Autodesk Fusion 360 part; units mm, degrees
(part 5 of 13)
  line L3550 (131.339, -140.663) -> (131.339, -140.663)
  line L3551 (130.416, -139.988) -> (130.432, -140.022)
  line L3552 (131.079, -140.585) -> (131.123, -140.605)
  line L3553 (129.684, -140.51) -> (129.684, -140.51)
  line L3554 (131.339, -140.663) -> (131.344, -140.664)
  line L3555 (130.303, -139.915) -> (130.371, -139.936)
  line L3556 (130.172, -140.022) -> (130.188, -139.988)
  line L3557 (128.804, -140.664) -> (129.032, -140.684)
  line L3558 (128.588, -140.606) -> (128.588, -140.606)
  line L3559 (130.732, -140.38) -> (130.733, -140.38)
  line L3560 (130.733, -140.38) -> (130.915, -140.508)
  line L3561 (131.572, -140.684) -> (131.8, -140.664)
  line L3562 (127.892, -140.022) -> (127.894, -140.027)
  line L3563 (128.192, -140.38) -> (128.192, -140.38)
  line L3564 (129.26, -140.664) -> (129.265, -140.663)
  line L3565 (127.149, -140.508) -> (127.331, -140.38)
  line L3566 (128.588, -140.606) -> (128.799, -140.663)
  line L3567 (130.732, -140.38) -> (130.732, -140.38)
  line L3568 (131.123, -140.605) -> (131.128, -140.606)
  line L3569 (135.315, -139.935) -> (135.383, -139.915)
  line L3570 (134.952, -140.38) -> (134.956, -140.377)
  line L3571 (132.911, -139.936) -> (132.956, -139.988)
  line L3572 (132.224, -140.51) -> (132.224, -140.51)
  line L3573 (133.106, -140.215) -> (133.268, -140.377)
  line L3574 (134.764, -140.51) -> (134.769, -140.508)
  line L3575 (132.578, -140.215) -> (132.71, -140.027)
  line L3576 (133.884, -140.664) -> (134.112, -140.684)
  line L3577 (130.235, -139.935) -> (130.303, -139.915)
  line L3578 (134.561, -140.605) -> (134.605, -140.585)
  line L3579 (132.972, -140.022) -> (132.972, -140.022)
  line L3580 (135.383, -139.915) -> (135.451, -139.936)
  line L3581 (134.34, -140.664) -> (134.345, -140.663)
  line L3582 (135.252, -140.022) -> (135.252, -140.022)
  line L3583 (132.712, -140.022) -> (132.728, -139.988)
  line L3584 (132.016, -140.606) -> (132.021, -140.605)
  line L3585 (130.038, -140.215) -> (130.17, -140.027)
  line L3586 (133.272, -140.38) -> (133.272, -140.38)
  line L3587 (131.128, -140.606) -> (131.339, -140.663)
  line L3588 (132.412, -140.38) -> (132.412, -140.38)
  line L3589 (132.016, -140.606) -> (132.016, -140.606)
  line L3590 (134.556, -140.606) -> (134.561, -140.605)
  line L3591 (134.956, -140.377) -> (135.118, -140.215)
  line L3592 (132.412, -140.38) -> (132.416, -140.377)
  line L3593 (134.764, -140.51) -> (134.764, -140.51)
  line L3594 (130.434, -140.027) -> (130.566, -140.215)
  line L3595 (133.273, -140.38) -> (133.455, -140.508)
  line L3596 (130.371, -139.936) -> (130.416, -139.988)
  line L3597 (133.455, -140.508) -> (133.46, -140.51)
  line L3598 (132.065, -140.585) -> (132.224, -140.51)
  line L3599 (133.272, -140.38) -> (133.273, -140.38)
  line L3600 (132.843, -139.915) -> (132.911, -139.936)
  line L3601 (133.619, -140.585) -> (133.663, -140.605)
  line L3602 (132.712, -140.022) -> (132.712, -140.022)
  line L3603 (130.17, -140.027) -> (130.172, -140.022)
  line L3604 (133.46, -140.51) -> (133.46, -140.51)
  line L3605 (132.411, -140.38) -> (132.412, -140.38)
  line L3606 (134.605, -140.585) -> (134.764, -140.51)
  line L3607 (132.974, -140.027) -> (133.106, -140.215)
  line L3608 (132.956, -139.988) -> (132.972, -140.022)
  line L3609 (134.951, -140.38) -> (134.952, -140.38)
  line L3610 (133.879, -140.663) -> (133.884, -140.664)
  line L3611 (134.769, -140.508) -> (134.951, -140.38)
  line L3612 (132.775, -139.935) -> (132.843, -139.915)
  line L3613 (132.021, -140.605) -> (132.065, -140.585)
  line L3614 (135.268, -139.988) -> (135.315, -139.935)
  line L3615 (133.668, -140.606) -> (133.879, -140.663)
  line L3616 (133.268, -140.377) -> (133.272, -140.38)
  line L3617 (135.252, -140.022) -> (135.268, -139.988)
  line L3618 (134.345, -140.663) -> (134.345, -140.663)
  line L3619 (132.972, -140.022) -> (132.974, -140.027)
  line L3620 (132.728, -139.988) -> (132.775, -139.935)
  line L3621 (132.416, -140.377) -> (132.578, -140.215)
  line L3622 (134.112, -140.684) -> (134.34, -140.664)
  line L3623 (135.451, -139.936) -> (135.496, -139.988)
  line L3624 (134.345, -140.663) -> (134.556, -140.606)
  line L3625 (130.728, -140.377) -> (130.732, -140.38)
  line L3626 (132.71, -140.027) -> (132.712, -140.022)
  line L3627 (131.805, -140.663) -> (131.805, -140.663)
  line L3628 (135.118, -140.215) -> (135.25, -140.027)
  line L3629 (132.229, -140.508) -> (132.411, -140.38)
  line L3630 (129.872, -140.38) -> (129.876, -140.377)
  line L3631 (132.224, -140.51) -> (132.229, -140.508)
  line L3632 (131.805, -140.663) -> (132.016, -140.606)
  line L3633 (137.309, -140.508) -> (137.491, -140.38)
  line L3634 (136.208, -140.606) -> (136.208, -140.606)
  line L3635 (139.425, -140.663) -> (139.425, -140.663)
  line L3636 (138.535, -140.508) -> (138.54, -140.51)
  line L3637 (137.658, -140.215) -> (137.79, -140.027)
  line L3638 (137.304, -140.51) -> (137.309, -140.508)
  line L3639 (137.101, -140.605) -> (137.145, -140.585)
  line L3640 (138.743, -140.605) -> (138.748, -140.606)
  line L3641 (136.159, -140.585) -> (136.203, -140.605)
  line L3642 (138.353, -140.38) -> (138.535, -140.508)
  line L3643 (136.208, -140.606) -> (136.419, -140.663)
  line L3644 (137.808, -139.988) -> (137.855, -139.935)
  line L3645 (137.991, -139.936) -> (138.036, -139.988)
  line L3646 (138.352, -140.38) -> (138.353, -140.38)
  line L3647 (138.352, -140.38) -> (138.352, -140.38)
  line L3648 (137.096, -140.606) -> (137.101, -140.605)
  line L3649 (137.492, -140.38) -> (137.496, -140.377)
  line L3650 (133.663, -140.605) -> (133.668, -140.606)
  line L3651 (136.419, -140.663) -> (136.419, -140.663)
  line L3652 (136.885, -140.663) -> (137.096, -140.606)
  line L3653 (138.964, -140.664) -> (139.192, -140.684)
  line L3654 (137.923, -139.915) -> (137.991, -139.936)
  line L3655 (138.699, -140.585) -> (138.743, -140.605)
  line L3656 (136.88, -140.664) -> (136.885, -140.663)
  line L3657 (135.812, -140.38) -> (135.812, -140.38)
  line L3658 (138.748, -140.606) -> (138.959, -140.663)
  line L3659 (137.491, -140.38) -> (137.492, -140.38)
  line L3660 (135.812, -140.38) -> (135.813, -140.38)
  line L3661 (138.959, -140.663) -> (138.959, -140.663)
  line L3662 (133.879, -140.663) -> (133.879, -140.663)
  line L3663 (135.995, -140.508) -> (136, -140.51)
  line L3664 (136, -140.51) -> (136, -140.51)
  line L3665 (136.203, -140.605) -> (136.208, -140.606)
  line L3666 (136.652, -140.684) -> (136.88, -140.664)
  line L3667 (137.145, -140.585) -> (137.304, -140.51)
  line L3668 (136.885, -140.663) -> (136.885, -140.663)
  line L3669 (137.492, -140.38) -> (137.492, -140.38)
  line L3670 (137.096, -140.606) -> (137.096, -140.606)
  line L3671 (137.79, -140.027) -> (137.792, -140.022)
  line L3672 (135.808, -140.377) -> (135.812, -140.38)
  line L3673 (137.304, -140.51) -> (137.304, -140.51)
  line L3674 (138.036, -139.988) -> (138.052, -140.022)
  line L3675 (135.646, -140.215) -> (135.808, -140.377)
  line L3676 (134.952, -140.38) -> (134.952, -140.38)
  line L3677 (136.419, -140.663) -> (136.424, -140.664)
  line L3678 (138.348, -140.377) -> (138.352, -140.38)
  line L3679 (139.42, -140.664) -> (139.425, -140.663)
  line L3680 (137.792, -140.022) -> (137.792, -140.022)
  line L3681 (135.813, -140.38) -> (135.995, -140.508)
  line L3682 (138.54, -140.51) -> (138.54, -140.51)
  line L3683 (135.25, -140.027) -> (135.252, -140.022)
  line L3684 (137.855, -139.935) -> (137.923, -139.915)
  line L3685 (134.556, -140.606) -> (134.556, -140.606)
  line L3686 (136.424, -140.664) -> (136.652, -140.684)
  line L3687 (139.425, -140.663) -> (139.636, -140.606)
  line L3688 (138.052, -140.022) -> (138.052, -140.022)
  line L3689 (133.46, -140.51) -> (133.619, -140.585)
  line L3690 (135.514, -140.027) -> (135.646, -140.215)
  line L3691 (139.192, -140.684) -> (139.42, -140.664)
  line L3692 (136, -140.51) -> (136.159, -140.585)
  line L3693 (135.512, -140.022) -> (135.514, -140.027)
  line L3694 (135.496, -139.988) -> (135.512, -140.022)
  line L3695 (133.668, -140.606) -> (133.668, -140.606)
  line L3696 (135.512, -140.022) -> (135.512, -140.022)
  line L3697 (142.576, -140.377) -> (142.738, -140.215)
  line L3698 (140.463, -139.915) -> (140.531, -139.936)
  line L3699 (140.031, -140.38) -> (140.032, -140.38)
  line L3700 (141.965, -140.663) -> (141.965, -140.663)
  line L3701 (140.395, -139.935) -> (140.463, -139.915)
  line L3702 (142.384, -140.51) -> (142.389, -140.508)
  line L3703 (142.176, -140.606) -> (142.181, -140.605)
  line L3704 (143.132, -140.022) -> (143.134, -140.027)
  line L3705 (140.332, -140.022) -> (140.348, -139.988)
  line L3706 (141.499, -140.663) -> (141.499, -140.663)
  line L3707 (142.87, -140.027) -> (142.872, -140.022)
  line L3708 (138.54, -140.51) -> (138.699, -140.585)
  line L3709 (140.892, -140.38) -> (140.892, -140.38)
  line L3710 (141.075, -140.508) -> (141.08, -140.51)
  line L3711 (139.844, -140.51) -> (139.844, -140.51)
  line L3712 (141.732, -140.684) -> (141.96, -140.664)
  line L3713 (139.636, -140.606) -> (139.641, -140.605)
  line L3714 (140.726, -140.215) -> (140.888, -140.377)
  line L3715 (141.08, -140.51) -> (141.239, -140.585)
  line L3716 (143.003, -139.915) -> (143.071, -139.936)
  line L3717 (140.332, -140.022) -> (140.332, -140.022)
  line L3718 (139.685, -140.585) -> (139.844, -140.51)
  line L3719 (140.893, -140.38) -> (141.075, -140.508)
  line L3720 (137.496, -140.377) -> (137.658, -140.215)
  line L3721 (140.594, -140.027) -> (140.726, -140.215)
  line L3722 (140.592, -140.022) -> (140.592, -140.022)
  line L3723 (139.849, -140.508) -> (140.031, -140.38)
  line L3724 (138.052, -140.022) -> (138.054, -140.027)
  line L3725 (141.08, -140.51) -> (141.08, -140.51)
  line L3726 (137.792, -140.022) -> (137.808, -139.988)
  line L3727 (139.641, -140.605) -> (139.685, -140.585)
  line L3728 (140.198, -140.215) -> (140.33, -140.027)
  line L3729 (140.032, -140.38) -> (140.032, -140.38)
  line L3730 (140.348, -139.988) -> (140.395, -139.935)
  line L3731 (141.288, -140.606) -> (141.499, -140.663)
  line L3732 (142.225, -140.585) -> (142.384, -140.51)
  line L3733 (140.531, -139.936) -> (140.576, -139.988)
  line L3734 (138.054, -140.027) -> (138.186, -140.215)
  line L3735 (140.33, -140.027) -> (140.332, -140.022)
  line L3736 (142.738, -140.215) -> (142.87, -140.027)
  line L3737 (142.888, -139.988) -> (142.935, -139.935)
  line L3738 (143.116, -139.988) -> (143.132, -140.022)
  line L3739 (143.132, -140.022) -> (143.132, -140.022)
  line L3740 (140.032, -140.38) -> (140.036, -140.377)
  line L3741 (141.283, -140.605) -> (141.288, -140.606)
  line L3742 (140.888, -140.377) -> (140.892, -140.38)
  line L3743 (141.504, -140.664) -> (141.732, -140.684)
  line L3744 (138.959, -140.663) -> (138.964, -140.664)
  line L3745 (138.748, -140.606) -> (138.748, -140.606)
  line L3746 (141.239, -140.585) -> (141.283, -140.605)
  line L3747 (140.036, -140.377) -> (140.198, -140.215)
  line L3748 (140.592, -140.022) -> (140.594, -140.027)
  line L3749 (139.844, -140.51) -> (139.849, -140.508)
  line L3750 (139.636, -140.606) -> (139.636, -140.606)
  line L3751 (142.935, -139.935) -> (143.003, -139.915)
  line L3752 (142.384, -140.51) -> (142.384, -140.51)
  line L3753 (138.186, -140.215) -> (138.348, -140.377)
  line L3754 (142.872, -140.022) -> (142.872, -140.022)
  line L3755 (140.576, -139.988) -> (140.592, -140.022)
  line L3756 (143.071, -139.936) -> (143.116, -139.988)
  line L3757 (141.965, -140.663) -> (142.176, -140.606)
  line L3758 (142.181, -140.605) -> (142.225, -140.585)
  line L3759 (140.892, -140.38) -> (140.893, -140.38)
  line L3760 (142.872, -140.022) -> (142.888, -139.988)
  line L3761 (143.828, -140.606) -> (143.828, -140.606)
  line L3762 (143.432, -140.38) -> (143.433, -140.38)
  line L3763 (143.823, -140.605) -> (143.828, -140.606)
  line L3764 (144.924, -140.51) -> (144.929, -140.508)
  line L3765 (145.428, -139.988) -> (145.475, -139.935)
  line L3766 (143.779, -140.585) -> (143.823, -140.605)
  line L3767 (145.968, -140.377) -> (145.972, -140.38)
  line L3768 (146.155, -140.508) -> (146.16, -140.51)
  line L3769 (143.266, -140.215) -> (143.428, -140.377)
  line L3770 (147.045, -140.663) -> (147.256, -140.606)
  line L3771 (144.5, -140.664) -> (144.505, -140.663)
  line L3772 (145.41, -140.027) -> (145.412, -140.022)
  line L3773 (144.929, -140.508) -> (145.111, -140.38)
  line L3774 (145.475, -139.935) -> (145.543, -139.915)
  line L3775 (146.368, -140.606) -> (146.579, -140.663)
  line L3776 (144.039, -140.663) -> (144.039, -140.663)
  line L3777 (143.432, -140.38) -> (143.432, -140.38)
  line L3778 (142.572, -140.38) -> (142.572, -140.38)
  line L3779 (145.278, -140.215) -> (145.41, -140.027)
  line L3780 (147.045, -140.663) -> (147.045, -140.663)
  line L3781 (145.543, -139.915) -> (145.611, -139.936)
  line L3782 (145.656, -139.988) -> (145.672, -140.022)
  line L3783 (146.16, -140.51) -> (146.16, -140.51)
  line L3784 (145.973, -140.38) -> (146.155, -140.508)
  line L3785 (143.428, -140.377) -> (143.432, -140.38)
  line L3786 (146.368, -140.606) -> (146.368, -140.606)
  line L3787 (144.924, -140.51) -> (144.924, -140.51)
  line L3788 (144.716, -140.606) -> (144.716, -140.606)
  line L3789 (143.62, -140.51) -> (143.779, -140.585)
  line L3790 (141.499, -140.663) -> (141.504, -140.664)
  line L3791 (146.319, -140.585) -> (146.363, -140.605)
  line L3792 (144.721, -140.605) -> (144.765, -140.585)
  line L3793 (145.116, -140.377) -> (145.278, -140.215)
  line L3794 (143.615, -140.508) -> (143.62, -140.51)
  line L3795 (143.828, -140.606) -> (144.039, -140.663)
  line L3796 (145.112, -140.38) -> (145.116, -140.377)
  line L3797 (144.765, -140.585) -> (144.924, -140.51)
  line L3798 (144.505, -140.663) -> (144.716, -140.606)
  line L3799 (146.584, -140.664) -> (146.812, -140.684)
  line L3800 (145.972, -140.38) -> (145.973, -140.38)
  line L3801 (143.433, -140.38) -> (143.615, -140.508)
  line L3802 (145.112, -140.38) -> (145.112, -140.38)
  line L3803 (144.505, -140.663) -> (144.505, -140.663)
  line L3804 (142.389, -140.508) -> (142.571, -140.38)
  line L3805 (143.134, -140.027) -> (143.266, -140.215)
  line L3806 (146.579, -140.663) -> (146.584, -140.664)
  line L3807 (144.039, -140.663) -> (144.044, -140.664)
  line L3808 (145.111, -140.38) -> (145.112, -140.38)
  line L3809 (144.716, -140.606) -> (144.721, -140.605)
  line L3810 (144.272, -140.684) -> (144.5, -140.664)
  line L3811 (142.572, -140.38) -> (142.576, -140.377)
  line L3812 (147.256, -140.606) -> (147.261, -140.605)
  line L3813 (142.571, -140.38) -> (142.572, -140.38)
  line L3814 (145.972, -140.38) -> (145.972, -140.38)
  line L3815 (145.674, -140.027) -> (145.806, -140.215)
  line L3816 (146.363, -140.605) -> (146.368, -140.606)
  line L3817 (142.176, -140.606) -> (142.176, -140.606)
  line L3818 (147.04, -140.664) -> (147.045, -140.663)
  line L3819 (146.579, -140.663) -> (146.579, -140.663)
  line L3820 (144.044, -140.664) -> (144.272, -140.684)
  line L3821 (141.288, -140.606) -> (141.288, -140.606)
  line L3822 (141.96, -140.664) -> (141.965, -140.663)
  line L3823 (143.62, -140.51) -> (143.62, -140.51)
  line L3824 (146.368, -138.135) -> (146.363, -138.136)
  line L3825 (148.046, -139.82) -> (148.106, -139.599)
  line L3826 (147.266, -138.139) -> (147.261, -138.136)
  line L3827 (146.358, -138.139) -> (146.358, -138.139)
  line L3828 (145.672, -140.022) -> (145.672, -140.022)
  line L3829 (146.16, -138.231) -> (146.16, -138.231)
  line L3830 (145.611, -139.936) -> (145.656, -139.988)
  line L3831 (147.656, -138.364) -> (147.652, -138.361)
  line L3832 (147.464, -138.231) -> (147.266, -138.139)
  line L3833 (145.656, -138.753) -> (145.609, -138.806)
  line L3834 (145.412, -140.022) -> (145.428, -139.988)
  line L3835 (147.952, -140.022) -> (147.952, -140.022)
  line L3836 (145.672, -138.719) -> (145.672, -138.719)
  line L3837 (147.952, -138.719) -> (147.952, -138.719)
  line L3838 (147.305, -140.585) -> (147.464, -140.51)
  line L3839 (148.106, -139.599) -> (148.125, -139.371)
  line L3840 (145.806, -138.526) -> (145.674, -138.714)
  line L3841 (147.987, -138.794) -> (147.952, -138.719)
  line L3842 (147.656, -140.377) -> (147.818, -140.215)
  line L3843 (145.412, -140.022) -> (145.412, -140.022)
  line L3844 (148.048, -138.927) -> (148.046, -138.921)
  line L3845 (146.16, -138.231) -> (146.155, -138.233)
  line L3846 (147.261, -140.605) -> (147.305, -140.585)
  line L3847 (146.16, -140.51) -> (146.319, -140.585)
  line L3848 (147.95, -140.027) -> (147.952, -140.022)
  line L3849 (147.266, -138.139) -> (147.266, -138.139)
  line L3850 (147.651, -140.38) -> (147.652, -140.38)
  line L3851 (147.261, -138.136) -> (147.256, -138.135)
  line L3852 (147.652, -138.361) -> (147.499, -138.254)
  line L3853 (146.812, -140.684) -> (147.04, -140.664)
  line L3854 (146.125, -138.254) -> (145.972, -138.361)
  line L3855 (147.469, -140.508) -> (147.651, -140.38)
  line L3856 (148.048, -138.927) -> (148.048, -138.927)
  line L3857 (148.106, -139.143) -> (148.104, -139.137)
  line L3858 (148.125, -139.371) -> (148.106, -139.143)
  line L3859 (147.818, -138.526) -> (147.656, -138.364)
  line L3860 (147.469, -138.233) -> (147.464, -138.231)
  line L3861 (147.464, -140.51) -> (147.464, -140.51)
  line L3862 (147.95, -138.714) -> (147.818, -138.526)
  line L3863 (145.972, -138.361) -> (145.968, -138.364)
  line L3864 (146.358, -138.139) -> (146.16, -138.231)
  line L3865 (146.155, -138.233) -> (146.125, -138.254)
  line L3866 (145.672, -138.719) -> (145.656, -138.753)
  line L3867 (145.672, -140.022) -> (145.674, -140.027)
  line L3868 (146.812, -138.057) -> (146.584, -138.077)
  line L3869 (147.045, -138.078) -> (147.04, -138.077)
  line L3870 (148.104, -139.137) -> (148.048, -138.927)
  line L3871 (145.806, -140.215) -> (145.968, -140.377)
  line L3872 (148.044, -139.825) -> (148.044, -139.825)
  line L3873 (145.674, -138.714) -> (145.672, -138.719)
  line L3874 (147.652, -138.361) -> (147.652, -138.361)
  line L3875 (147.952, -138.719) -> (147.95, -138.714)
  line L3876 (147.818, -140.215) -> (147.95, -140.027)
  line L3877 (147.464, -140.51) -> (147.469, -140.508)
  line L3878 (148.044, -139.825) -> (148.046, -139.82)
  line L3879 (147.256, -138.135) -> (147.256, -138.135)
  line L3880 (146.363, -138.136) -> (146.358, -138.139)
  line L3881 (147.952, -140.022) -> (148.044, -139.825)
  line L3882 (148.046, -138.921) -> (147.987, -138.794)
  line L3883 (147.652, -140.38) -> (147.652, -140.38)
  line L3884 (147.256, -140.606) -> (147.256, -140.606)
  line L3885 (145.968, -138.364) -> (145.806, -138.526)
  line L3886 (147.499, -138.254) -> (147.469, -138.233)
  line L3887 (147.652, -140.38) -> (147.656, -140.377)
  line L3888 (106.95, -138.191) -> (106.756, -138.084)
  line L3889 (146.368, -138.135) -> (146.368, -138.135)
  line L3890 (106.751, -138.081) -> (106.746, -138.08)
  line L3891 (105.844, -137.996) -> (105.624, -138.068)
  line L3892 (106.31, -137.964) -> (106.305, -137.964)
  line L3893 (145.428, -138.753) -> (145.412, -138.719)
  line L3894 (144.716, -138.135) -> (144.716, -138.135)
  line L3895 (144.924, -138.231) -> (144.924, -138.231)
  line L3896 (144.505, -138.078) -> (144.5, -138.077)
  line L3897 (144.721, -138.136) -> (144.716, -138.135)
  line L3898 (145.412, -138.719) -> (145.412, -138.719)
  line L3899 (106.528, -138.003) -> (106.31, -137.964)
  line L3900 (105.624, -138.068) -> (105.62, -138.07)
  line L3901 (107.161, -138.364) -> (107.136, -138.337)
  line L3902 (145.473, -138.805) -> (145.428, -138.753)
  line L3903 (106.31, -137.964) -> (106.31, -137.964)
  line L3904 (147.045, -138.078) -> (147.045, -138.078)
  line L3905 (145.112, -138.361) -> (144.959, -138.254)
  line L3906 (145.278, -138.526) -> (145.116, -138.364)
  line L3907 (144.039, -138.078) -> (144.039, -138.078)
  line L3908 (146.579, -138.078) -> (146.579, -138.078)
  line L3909 (146.579, -138.078) -> (146.368, -138.135)
  line L3910 (145.609, -138.806) -> (145.541, -138.826)
  line L3911 (144.726, -138.139) -> (144.721, -138.136)
  line L3912 (105.471, -138.147) -> (105.419, -138.175)
  line L3913 (106.746, -138.08) -> (106.538, -138.006)
  line L3914 (106.538, -138.006) -> (106.533, -138.004)
  line L3915 (144.272, -138.057) -> (144.044, -138.077)
  line L3916 (105.419, -138.175) -> (105.415, -138.178)
  line L3917 (144.716, -138.135) -> (144.505, -138.078)
  line L3918 (145.541, -138.826) -> (145.473, -138.805)
  line L3919 (106.756, -138.084) -> (106.751, -138.081)
  line L3920 (106.95, -138.191) -> (106.95, -138.191)
  line L3921 (106.958, -138.197) -> (106.958, -138.197)
  line L3922 (106.538, -138.006) -> (106.538, -138.006)
  line L3923 (144.044, -138.077) -> (144.039, -138.078)
  line L3924 (106.958, -138.197) -> (106.954, -138.193)
  line L3925 (106.073, -137.961) -> (105.844, -137.996)
  line L3926 (145.41, -138.714) -> (145.278, -138.526)
  line L3927 (106.746, -138.08) -> (106.746, -138.08)
  line L3928 (107.132, -138.334) -> (107.132, -138.334)
  line L3929 (107.132, -138.334) -> (106.958, -138.197)
  line L3930 (106.533, -138.004) -> (106.528, -138.003)
  line L3931 (144.959, -138.254) -> (144.929, -138.233)
  line L3932 (106.954, -138.193) -> (106.95, -138.191)
  line L3933 (144.924, -138.231) -> (144.726, -138.139)
  line L3934 (147.464, -138.231) -> (147.464, -138.231)
  line L3935 (145.972, -138.361) -> (145.972, -138.361)
  line L3936 (147.04, -138.077) -> (146.812, -138.057)
  line L3937 (146.584, -138.077) -> (146.579, -138.078)
  line L3938 (144.505, -138.078) -> (144.505, -138.078)
  line L3939 (106.305, -137.964) -> (106.232, -137.963)
  line L3940 (145.116, -138.364) -> (145.112, -138.361)
  line L3941 (144.5, -138.077) -> (144.272, -138.057)
  line L3942 (145.412, -138.719) -> (145.41, -138.714)
  line L3943 (144.929, -138.233) -> (144.924, -138.231)
  line L3944 (144.726, -138.139) -> (144.726, -138.139)
  line L3945 (147.256, -138.135) -> (147.045, -138.078)
  line L3946 (106.528, -138.003) -> (106.528, -138.003)
  line L3947 (106.232, -137.963) -> (106.079, -137.961)
  line L3948 (106.079, -137.961) -> (106.079, -137.961)
  line L3949 (105.62, -138.07) -> (105.62, -138.07)
  line L3950 (145.112, -138.361) -> (145.112, -138.361)
  line L3951 (106.756, -138.084) -> (106.756, -138.084)
  line L3952 (140.594, -138.714) -> (140.592, -138.719)
  line L3953 (143.823, -138.136) -> (143.818, -138.139)
  line L3954 (140.892, -138.361) -> (140.892, -138.361)
  line L3955 (141.96, -138.077) -> (141.732, -138.057)
  line L3956 (142.181, -138.136) -> (142.176, -138.135)
  line L3957 (142.87, -138.714) -> (142.738, -138.526)
  line L3958 (143.432, -138.361) -> (143.432, -138.361)
  line L3959 (143.585, -138.254) -> (143.432, -138.361)
  line L3960 (143.828, -138.135) -> (143.828, -138.135)
  line L3961 (140.888, -138.364) -> (140.726, -138.526)
  line L3962 (142.572, -138.361) -> (142.419, -138.254)
  line L3963 (142.576, -138.364) -> (142.572, -138.361)
  line L3964 (142.176, -138.135) -> (142.176, -138.135)
  line L3965 (140.592, -138.719) -> (140.592, -138.719)
  line L3966 (143.428, -138.364) -> (143.266, -138.526)
  line L3967 (141.965, -138.078) -> (141.965, -138.078)
  line L3968 (143.615, -138.233) -> (143.585, -138.254)
  line L3969 (107.136, -138.337) -> (107.132, -138.334)
  line L3970 (144.039, -138.078) -> (143.828, -138.135)
  line L3971 (142.888, -138.753) -> (142.872, -138.719)
  line L3972 (142.933, -138.805) -> (142.888, -138.753)
  line L3973 (142.872, -138.719) -> (142.872, -138.719)
  line L3974 (141.278, -138.139) -> (141.278, -138.139)
  line L3975 (143.116, -138.753) -> (143.069, -138.806)
  line L3976 (143.828, -138.135) -> (143.823, -138.136)
  line L3977 (142.186, -138.139) -> (142.186, -138.139)
  line L3978 (141.288, -138.135) -> (141.288, -138.135)
  line L3979 (142.872, -138.719) -> (142.87, -138.714)
  line L3980 (140.726, -138.526) -> (140.594, -138.714)
  line L3981 (143.62, -138.231) -> (143.615, -138.233)
  line L3982 (142.572, -138.361) -> (142.572, -138.361)
  line L3983 (142.186, -138.139) -> (142.181, -138.136)
  line L3984 (140.892, -138.361) -> (140.888, -138.364)
  line L3985 (141.732, -138.057) -> (141.504, -138.077)
  line L3986 (141.504, -138.077) -> (141.499, -138.078)
  line L3987 (142.389, -138.233) -> (142.384, -138.231)
  line L3988 (141.08, -138.231) -> (141.08, -138.231)
  line L3989 (140.592, -138.719) -> (140.576, -138.753)
  line L3990 (142.738, -138.526) -> (142.576, -138.364)
  line L3991 (106.079, -137.961) -> (106.073, -137.961)
  line L3992 (141.075, -138.233) -> (141.045, -138.254)
  line L3993 (141.499, -138.078) -> (141.288, -138.135)
  line L3994 (140.576, -138.753) -> (140.529, -138.806)
  line L3995 (141.045, -138.254) -> (140.892, -138.361)
  line L3996 (141.283, -138.136) -> (141.278, -138.139)
  line L3997 (143.132, -138.719) -> (143.132, -138.719)
  line L3998 (143.266, -138.526) -> (143.134, -138.714)
  line L3999 (142.384, -138.231) -> (142.384, -138.231)
  line L4000 (143.001, -138.826) -> (142.933, -138.805)
  line L4001 (143.132, -138.719) -> (143.116, -138.753)
  line L4002 (143.818, -138.139) -> (143.818, -138.139)
  line L4003 (142.176, -138.135) -> (141.965, -138.078)
  line L4004 (105.62, -138.07) -> (105.471, -138.147)
  line L4005 (143.432, -138.361) -> (143.428, -138.364)
  line L4006 (143.069, -138.806) -> (143.001, -138.826)
  line L4007 (143.818, -138.139) -> (143.62, -138.231)
  line L4008 (142.419, -138.254) -> (142.389, -138.233)
  line L4009 (143.134, -138.714) -> (143.132, -138.719)
  line L4010 (143.62, -138.231) -> (143.62, -138.231)
  line L4011 (141.965, -138.078) -> (141.96, -138.077)
  line L4012 (141.499, -138.078) -> (141.499, -138.078)
  line L4013 (141.278, -138.139) -> (141.08, -138.231)
  line L4014 (142.384, -138.231) -> (142.186, -138.139)
  line L4015 (141.08, -138.231) -> (141.075, -138.233)
  line L4016 (140.198, -138.526) -> (140.036, -138.364)
  line L4017 (140.032, -138.361) -> (140.032, -138.361)
  line L4018 (139.879, -138.254) -> (139.849, -138.233)
  line L4019 (138.738, -138.139) -> (138.738, -138.139)
  line L4020 (138.959, -138.078) -> (138.748, -138.135)
  line L4021 (139.425, -138.078) -> (139.425, -138.078)
  line L4022 (140.348, -138.753) -> (140.332, -138.719)
  line L4023 (140.032, -138.361) -> (139.879, -138.254)
  line L4024 (139.646, -138.139) -> (139.641, -138.136)
  line L4025 (138.743, -138.136) -> (138.738, -138.139)
  line L4026 (140.33, -138.714) -> (140.198, -138.526)
  line L4027 (139.192, -138.057) -> (138.964, -138.077)
  line L4028 (139.42, -138.077) -> (139.192, -138.057)
  line L4029 (140.332, -138.719) -> (140.332, -138.719)
  line L4030 (140.529, -138.806) -> (140.461, -138.826)
  line L4031 (139.849, -138.233) -> (139.844, -138.231)
  line L4032 (139.641, -138.136) -> (139.636, -138.135)
  line L4033 (139.636, -138.135) -> (139.636, -138.135)
  line L4034 (138.54, -138.231) -> (138.535, -138.233)
  line L4035 (139.844, -138.231) -> (139.646, -138.139)
  line L4036 (138.964, -138.077) -> (138.959, -138.078)
  line L4037 (138.959, -138.078) -> (138.959, -138.078)
  line L4038 (138.54, -138.231) -> (138.54, -138.231)
  line L4039 (140.461, -138.826) -> (140.393, -138.805)
  line L4040 (138.748, -138.135) -> (138.748, -138.135)
  line L4041 (141.288, -138.135) -> (141.283, -138.136)
  line L4042 (138.748, -138.135) -> (138.743, -138.136)
  line L4043 (140.332, -138.719) -> (140.33, -138.714)
  line L4044 (140.393, -138.805) -> (140.348, -138.753)
  line L4045 (137.79, -138.714) -> (137.658, -138.526)
  line L4046 (138.052, -138.719) -> (138.036, -138.753)
  line L4047 (137.339, -138.254) -> (137.309, -138.233)
  line L4048 (138.505, -138.254) -> (138.352, -138.361)
  line L4049 (138.054, -138.714) -> (138.052, -138.719)
  line L4050 (138.186, -138.526) -> (138.054, -138.714)
  line L4051 (135.812, -138.361) -> (135.808, -138.364)
  line L4052 (137.096, -138.135) -> (136.885, -138.078)
  line L4053 (140.036, -138.364) -> (140.032, -138.361)
  line L4054 (137.853, -138.805) -> (137.808, -138.753)
  line L4055 (139.844, -138.231) -> (139.844, -138.231)
  line L4056 (137.808, -138.753) -> (137.792, -138.719)
  line L4057 (137.106, -138.139) -> (137.101, -138.136)
  line L4058 (137.496, -138.364) -> (137.492, -138.361)
  line L4059 (137.989, -138.806) -> (137.921, -138.826)
  line L4060 (137.304, -138.231) -> (137.106, -138.139)
  line L4061 (138.036, -138.753) -> (137.989, -138.806)
  line L4062 (138.352, -138.361) -> (138.352, -138.361)
  line L4063 (138.738, -138.139) -> (138.54, -138.231)
  line L4064 (136.885, -138.078) -> (136.885, -138.078)
  line L4065 (137.792, -138.719) -> (137.792, -138.719)
  line L4066 (138.352, -138.361) -> (138.348, -138.364)
  line L4067 (139.646, -138.139) -> (139.646, -138.139)
  line L4068 (139.425, -138.078) -> (139.42, -138.077)
  line L4069 (137.096, -138.135) -> (137.096, -138.135)
  line L4070 (137.658, -138.526) -> (137.496, -138.364)
  line L4071 (138.535, -138.233) -> (138.505, -138.254)
  line L4072 (137.921, -138.826) -> (137.853, -138.805)
  line L4073 (138.052, -138.719) -> (138.052, -138.719)
  line L4074 (137.101, -138.136) -> (137.096, -138.135)
  line L4075 (137.792, -138.719) -> (137.79, -138.714)
  line L4076 (137.106, -138.139) -> (137.106, -138.139)
  line L4077 (137.492, -138.361) -> (137.492, -138.361)
  line L4078 (137.309, -138.233) -> (137.304, -138.231)
  line L4079 (137.492, -138.361) -> (137.339, -138.254)
  line L4080 (137.304, -138.231) -> (137.304, -138.231)
  line L4081 (139.636, -138.135) -> (139.425, -138.078)
  line L4082 (136.885, -138.078) -> (136.88, -138.077)
  line L4083 (138.348, -138.364) -> (138.186, -138.526)
  line L4084 (134.566, -138.139) -> (134.566, -138.139)
  line L4085 (132.972, -138.719) -> (132.972, -138.719)
  line L4086 (136.198, -138.139) -> (136, -138.231)
  line L4087 (135.965, -138.254) -> (135.812, -138.361)
  line L4088 (136.419, -138.078) -> (136.208, -138.135)
  line L4089 (136.652, -138.057) -> (136.424, -138.077)
  line L4090 (135.808, -138.364) -> (135.646, -138.526)
  line L4091 (135.646, -138.526) -> (135.514, -138.714)
  line L4092 (135.25, -138.714) -> (135.118, -138.526)
  line L4093 (136.424, -138.077) -> (136.419, -138.078)
  line L4094 (135.995, -138.233) -> (135.965, -138.254)
  line L4095 (135.496, -138.753) -> (135.449, -138.806)
  line L4096 (135.252, -138.719) -> (135.25, -138.714)
  line L4097 (133.46, -138.231) -> (133.455, -138.233)
  line L4098 (133.272, -138.361) -> (133.268, -138.364)
  line L4099 (134.561, -138.136) -> (134.556, -138.135)
  line L4100 (134.799, -138.254) -> (134.769, -138.233)
  line L4101 (134.345, -138.078) -> (134.34, -138.077)
  line L4102 (136.88, -138.077) -> (136.652, -138.057)
  line L4103 (135.252, -138.719) -> (135.252, -138.719)
  line L4104 (136.419, -138.078) -> (136.419, -138.078)
  line L4105 (136.208, -138.135) -> (136.203, -138.136)
  line L4106 (135.118, -138.526) -> (134.956, -138.364)
  line L4107 (134.956, -138.364) -> (134.952, -138.361)
  line L4108 (134.952, -138.361) -> (134.952, -138.361)
  line L4109 (135.512, -138.719) -> (135.512, -138.719)
  line L4110 (133.668, -138.135) -> (133.663, -138.136)
  line L4111 (133.425, -138.254) -> (133.272, -138.361)
  line L4112 (134.952, -138.361) -> (134.799, -138.254)
  line L4113 (133.455, -138.233) -> (133.425, -138.254)
  line L4114 (133.106, -138.526) -> (132.974, -138.714)
  line L4115 (135.313, -138.805) -> (135.268, -138.753)
  line L4116 (136.203, -138.136) -> (136.198, -138.139)
  line L4117 (136.208, -138.135) -> (136.208, -138.135)
  line L4118 (133.46, -138.231) -> (133.46, -138.231)
  line L4119 (135.268, -138.753) -> (135.252, -138.719)
  line L4120 (134.566, -138.139) -> (134.561, -138.136)
  line L4121 (133.658, -138.139) -> (133.658, -138.139)
  line L4122 (134.112, -138.057) -> (133.884, -138.077)
  line L4123 (135.449, -138.806) -> (135.381, -138.826)
  line L4124 (136, -138.231) -> (135.995, -138.233)
  line L4125 (135.812, -138.361) -> (135.812, -138.361)
  line L4126 (136, -138.231) -> (136, -138.231)
  line L4127 (133.658, -138.139) -> (133.46, -138.231)
  line L4128 (135.514, -138.714) -> (135.512, -138.719)
  line L4129 (136.198, -138.139) -> (136.198, -138.139)
  line L4130 (135.381, -138.826) -> (135.313, -138.805)
  line L4131 (135.512, -138.719) -> (135.496, -138.753)
  line L4132 (134.769, -138.233) -> (134.764, -138.231)
  line L4133 (130.369, -138.806) -> (130.301, -138.826)
  line L4134 (132.412, -138.361) -> (132.412, -138.361)
  line L4135 (132.71, -138.714) -> (132.578, -138.526)
  line L4136 (129.684, -138.231) -> (129.486, -138.139)
  line L4137 (134.345, -138.078) -> (134.345, -138.078)
  line L4138 (132.016, -138.135) -> (132.016, -138.135)
  line L4139 (132.259, -138.254) -> (132.229, -138.233)
  line L4140 (131.128, -138.135) -> (131.128, -138.135)
  line L4141 (130.172, -138.719) -> (130.17, -138.714)
  line L4142 (130.038, -138.526) -> (129.876, -138.364)
  line L4143 (132.909, -138.806) -> (132.841, -138.826)
  line L4144 (129.486, -138.139) -> (129.486, -138.139)
  line L4145 (133.884, -138.077) -> (133.879, -138.078)
  line L4146 (133.663, -138.136) -> (133.658, -138.139)
  line L4147 (132.956, -138.753) -> (132.909, -138.806)
  line L4148 (129.876, -138.364) -> (129.872, -138.361)
  line L4149 (132.728, -138.753) -> (132.712, -138.719)
  line L4150 (134.764, -138.231) -> (134.566, -138.139)
  line L4151 (134.764, -138.231) -> (134.764, -138.231)
  line L4152 (134.556, -138.135) -> (134.345, -138.078)
  line L4153 (132.026, -138.139) -> (132.021, -138.136)
  line L4154 (133.268, -138.364) -> (133.106, -138.526)
  line L4155 (131.128, -138.135) -> (131.123, -138.136)
  line L4156 (134.556, -138.135) -> (134.556, -138.135)
  line L4157 (131.123, -138.136) -> (131.118, -138.139)
  line L4158 (132.972, -138.719) -> (132.956, -138.753)
  line L4159 (133.272, -138.361) -> (133.272, -138.361)
  line L4160 (132.841, -138.826) -> (132.773, -138.805)
  line L4161 (132.224, -138.231) -> (132.026, -138.139)
  line L4162 (132.021, -138.136) -> (132.016, -138.135)
  line L4163 (132.712, -138.719) -> (132.71, -138.714)
  line L4164 (131.8, -138.077) -> (131.572, -138.057)
  line L4165 (133.668, -138.135) -> (133.668, -138.135)
  line L4166 (133.879, -138.078) -> (133.668, -138.135)
  line L4167 (131.339, -138.078) -> (131.339, -138.078)
  line L4168 (131.805, -138.078) -> (131.805, -138.078)
  line L4169 (132.016, -138.135) -> (131.805, -138.078)
  line L4170 (131.339, -138.078) -> (131.128, -138.135)
  line L4171 (130.301, -138.826) -> (130.233, -138.805)
  line L4172 (131.805, -138.078) -> (131.8, -138.077)
  line L4173 (129.872, -138.361) -> (129.872, -138.361)
  line L4174 (132.578, -138.526) -> (132.416, -138.364)
  line L4175 (132.712, -138.719) -> (132.712, -138.719)
  line L4176 (131.572, -138.057) -> (131.344, -138.077)
  line L4177 (132.974, -138.714) -> (132.972, -138.719)
  line L4178 (132.229, -138.233) -> (132.224, -138.231)
  line L4179 (132.773, -138.805) -> (132.728, -138.753)
  line L4180 (131.344, -138.077) -> (131.339, -138.078)
  line L4181 (133.879, -138.078) -> (133.879, -138.078)
  line L4182 (134.34, -138.077) -> (134.112, -138.057)
  line L4183 (132.224, -138.231) -> (132.224, -138.231)
  line L4184 (132.026, -138.139) -> (132.026, -138.139)
  line L4185 (130.434, -138.714) -> (130.432, -138.719)
  line L4186 (132.416, -138.364) -> (132.412, -138.361)
  line L4187 (131.118, -138.139) -> (131.118, -138.139)
  line L4188 (129.684, -138.231) -> (129.684, -138.231)
  line L4189 (130.233, -138.805) -> (130.188, -138.753)
  line L4190 (131.118, -138.139) -> (130.92, -138.231)
  line L4191 (132.412, -138.361) -> (132.259, -138.254)
  line L4192 (130.416, -138.753) -> (130.369, -138.806)
  line L4193 (149.275, -96.9044) -> (149.295, -97.028)
  line L4194 (149.262, -97.9272) -> (149.263, -97.9874)
  line L4195 (149.264, -98.0232) -> (149.264, -98.0233)
  line L4196 (149.263, -97.9913) -> (149.263, -98.0193)
  line L4197 (149.263, -97.1746) -> (149.263, -97.9006)
  line L4198 (149.131, -96.0386) -> (149.167, -96.078)
  line L4199 (149.264, -98.0233) -> (149.265, -98.0351)
  line L4200 (149.263, -97.9006) -> (149.263, -97.9118)
  line L4201 (149.275, -97.1516) -> (149.263, -97.1746)
  line L4202 (149.265, -98.0351) -> (149.266, -98.0793)
  line L4203 (149.315, -98.2398) -> (149.321, -98.2504)
  line L4204 (149.791, -101.311) -> (149.737, -101.357)
  line L4205 (149.271, -98.0951) -> (149.272, -98.0987)
  line L4206 (149.299, -98.1905) -> (149.311, -98.233)
  line L4207 (149.315, -98.2398) -> (149.315, -98.2398)
  line L4208 (149.321, -98.2504) -> (149.33, -98.2682)
  line L4209 (149.295, -98.1793) -> (149.299, -98.1905)
  line L4210 (149.279, -98.1382) -> (149.281, -98.1456)
  line L4211 (149.266, -98.0793) -> (149.271, -98.0951)
  line L4212 (149.263, -96.2448) -> (149.263, -96.8814)
  line L4213 (148.786, -95.825) -> (148.676, -95.7145)
  line L4214 (148.92, -96.2914) -> (148.935, -96.2869)
  line L4215 (148.43, -96.2914) -> (148.92, -96.2914)
  line L4216 (149.011, -95.573) -> (149.026, -95.7178)
  line L4217 (150.213, -94.7069) -> (150.213, -94.7069)
  line L4218 (149.448, -94.7967) -> (149.313, -94.8942)
  line L4219 (150.381, -94.7819) -> (150.375, -94.7792)
  line L4220 (149.474, -94.7792) -> (149.468, -94.7819)
  line L4221 (149.031, -95.7627) -> (149.018, -95.8326)
  line L4222 (149.186, -95.0361) -> (149.09, -95.2015)
  line L4223 (149.262, -96.2245) -> (149.263, -96.2448)
  line L4224 (149.026, -95.7178) -> (149.031, -95.7627)
  line L4225 (148.516, -95.6181) -> (148.367, -95.5711)
  line L4226 (148.834, -95.8792) -> (148.798, -95.8412)
  line L4227 (148.933, -96.1525) -> (148.946, -96.0829)
  line L4228 (149.231, -96.1605) -> (149.262, -96.2245)
  line L4229 (148.935, -96.2869) -> (148.937, -96.2855)
  line L4230 (148.43, -96.2704) -> (148.43, -96.2914)
  line L4231 (149.031, -95.3831) -> (149.011, -95.573)
  line L4232 (148.937, -96.2855) -> (148.938, -96.2779)
  line L4233 (149.186, -96.11) -> (149.224, -96.1525)
  line L4234 (148.372, -96.129) -> (148.415, -96.1939)
  line L4235 (148.415, -96.1939) -> (148.43, -96.2704)
  line L4236 (148.299, -95.5635) -> (148.287, -95.5669)
  line L4237 (148.901, -95.9018) -> (148.834, -95.8792)
  line L4238 (148.284, -96.0811) -> (148.307, -96.0856)
  line L4239 (148.798, -95.8412) -> (148.795, -95.8368)
  line L4240 (150.207, -94.7042) -> (150.114, -94.6844)
  line L4241 (149.09, -95.2015) -> (149.031, -95.3831)
  line L4242 (149.263, -97.9118) -> (149.261, -97.9193)
  line L4243 (148.676, -95.7145) -> (148.664, -95.7052)
  line L4244 (148.995, -96.0317) -> (149.064, -96.0152)
  line L4245 (150.387, -94.7858) -> (150.387, -94.7858)
  line L4246 (149.295, -97.028) -> (149.275, -97.1516)
  line L4247 (148.287, -95.5669) -> (148.286, -95.5683)
  line L4248 (149.262, -97.9272) -> (149.262, -97.9272)
  line L4249 (149.064, -96.0152) -> (149.131, -96.0386)
  line L4250 (149.018, -95.8326) -> (148.97, -95.8844)
  line L4251 (148.795, -95.8368) -> (148.786, -95.825)
  line L4252 (150.402, -94.7967) -> (150.387, -94.7858)
  line L4253 (149.463, -94.7858) -> (149.448, -94.7967)
  line L4254 (148.664, -95.7052) -> (148.53, -95.6243)
  line L4255 (148.367, -95.5711) -> (148.354, -95.5685)
  line L4256 (148.354, -95.5685) -> (148.299, -95.5635)
  line L4257 (148.97, -95.8844) -> (148.901, -95.9018)
  line L4258 (148.53, -95.6243) -> (148.516, -95.6181)
  line L4259 (149.224, -96.1525) -> (149.231, -96.1605)
  line L4260 (148.946, -96.0829) -> (148.995, -96.0317)
  line L4261 (148.286, -95.5683) -> (148.284, -95.5759)
  line L4262 (148.307, -96.0856) -> (148.372, -96.129)
  line L4263 (149.263, -96.8814) -> (149.275, -96.9044)
  line L4264 (148.284, -95.5759) -> (148.284, -96.0811)
  line L4265 (148.938, -96.2779) -> (148.938, -96.2167)
  line L4266 (149.261, -97.9193) -> (149.262, -97.9272)
  line L4267 (148.938, -96.2167) -> (148.938, -96.2109)
  line L4268 (149.263, -97.9874) -> (149.263, -97.9913)
  line L4269 (149.263, -98.0193) -> (149.264, -98.0232)
  line L4270 (148.938, -96.2109) -> (148.933, -96.1525)
  line L4271 (149.167, -96.078) -> (149.186, -96.11)
  line L4272 (149.264, -98.0232) -> (149.264, -98.0232)
  line L4273 (126.511, -110.725) -> (126.422, -110.814)
  line L4274 (126.318, -108.058) -> (126.318, -110.113)
  line L4275 (125.787, -110.49) -> (125.807, -110.366)
  line L4276 (116.587, -110.012) -> (116.581, -110.017)
  line L4277 (126.299, -107.993) -> (126.303, -107.998)
  line L4278 (125.939, -102.231) -> (125.94, -102.225)
  line L4279 (126.068, -108.11) -> (125.972, -108.013)
  line L4280 (126.303, -107.998) -> (126.31, -108.028)
  line L4281 (116.592, -110.006) -> (116.587, -110.012)
  line L4282 (115.998, -108.184) -> (116.003, -108.183)
  line L4283 (116.593, -108.848) -> (116.593, -109.998)
  line L4284 (116.498, -108.655) -> (116.499, -108.658)
  line L4285 (126.064, -110.11) -> (126.068, -110.109)
  line L4286 (126.311, -110.87) -> (126.187, -110.89)
  line L4287 (116.495, -108.652) -> (116.498, -108.655)
  line L4288 (116.587, -108.834) -> (116.592, -108.841)
  line L4289 (126.187, -110.89) -> (126.064, -110.87)
  line L4290 (116.573, -108.828) -> (116.581, -108.83)
  line L4291 (116.482, -108.634) -> (116.495, -108.652)
  line L4292 (129.772, -98.3722) -> (129.772, -96.9696)
  line L4293 (116.593, -109.998) -> (116.592, -110.006)
  line L4294 (126.31, -108.028) -> (126.318, -108.058)
  line L4295 (125.972, -102.172) -> (129.772, -98.3722)
  line L4296 (116.518, -108.722) -> (116.518, -108.828)
  line L4297 (125.957, -102.199) -> (125.972, -102.172)
  line L4298 (116.006, -108.185) -> (116.012, -108.186)
  line L4299 (125.938, -102.234) -> (125.939, -102.231)
  line L4300 (116.503, -108.663) -> (116.51, -108.693)
  line L4301 (125.955, -107.992) -> (125.954, -107.989)
  line L4302 (125.958, -107.995) -> (125.955, -107.992)
  line L4303 (116.581, -108.83) -> (116.587, -108.834)
  line L4304 (126.587, -110.49) -> (126.568, -110.614)
  line L4305 (125.938, -102.238) -> (125.938, -102.234)
  line L4306 (125.94, -102.225) -> (125.957, -102.199)
  line L4307 (125.952, -110.814) -> (125.864, -110.725)
  line L4308 (125.807, -110.366) -> (125.864, -110.255)
  line L4309 (116.518, -108.828) -> (116.573, -108.828)
  line L4310 (116.038, -108.202) -> (116.065, -108.217)
  line L4311 (116.065, -108.217) -> (116.482, -108.634)
  line L4312 (116.581, -110.017) -> (116.573, -110.018)
  line L4313 (116.592, -108.841) -> (116.593, -108.848)
  line L4314 (126.568, -110.366) -> (126.587, -110.49)
  line L4315 (125.935, -107.925) -> (125.935, -102.26)
  line L4316 (112.449, -109.754) -> (112.573, -109.734)
  line L4317 (115.577, -108.34) -> (115.7, -108.217)
  line L4318 (115.721, -108.2) -> (115.723, -108.2)
  line L4319 (112.696, -110.515) -> (112.573, -110.534)
  line L4320 (112.338, -109.811) -> (112.449, -109.754)
  line L4321 (115.577, -108.694) -> (115.577, -109.767)
  line L4322 (116.199, -110.012) -> (116.195, -110.006)
  line L4323 (116.195, -108.841) -> (116.199, -108.834)
  line L4324 (116.213, -108.828) -> (116.268, -108.828)
  line L4325 (115.925, -108.431) -> (115.84, -108.431)
  line L4326 (112.953, -110.258) -> (112.896, -110.37)
  line L4327 (116.499, -108.658) -> (116.503, -108.663)
  line L4328 (116.268, -108.828) -> (116.268, -108.774)
  line L4329 (116.51, -108.693) -> (116.518, -108.722)
  line L4330 (114.577, -109.617) -> (114.277, -109.617)
  line L4331 (116.213, -110.018) -> (116.206, -110.017)
  line L4332 (115.577, -109.767) -> (114.577, -109.767)
  line L4333 (116.199, -108.834) -> (116.206, -108.83)
  line L4334 (116.193, -108.848) -> (116.195, -108.841)
  line L4335 (112.449, -110.515) -> (112.338, -110.458)
  line L4336 (116.206, -110.017) -> (116.199, -110.012)
  line L4337 (114.277, -109.617) -> (114.277, -109.767)
  line L4338 (116.195, -110.006) -> (116.193, -109.998)
  line L4339 (116.003, -108.183) -> (116.006, -108.185)
  line L4340 (125.935, -102.26) -> (125.938, -102.238)
  line L4341 (116.268, -108.774) -> (115.925, -108.431)
  line L4342 (112.896, -110.37) -> (112.808, -110.458)
  line L4343 (113.277, -109.767) -> (113.277, -109.607)
  line L4344 (114.577, -109.767) -> (114.577, -109.617)
  line L4345 (114.277, -109.767) -> (113.277, -109.767)
  line L4346 (112.573, -110.534) -> (112.449, -110.515)
  line L4347 (116.573, -110.018) -> (116.213, -110.018)
  line L4348 (112.808, -110.458) -> (112.696, -110.515)
  line L4349 (116.206, -108.83) -> (116.213, -108.828)
  line L4350 (112.973, -110.134) -> (112.953, -110.258)
  line L4351 (116.012, -108.186) -> (116.038, -108.202)
  line L4352 (116.193, -109.998) -> (116.193, -108.848)
  line L4353 (115.84, -108.431) -> (115.577, -108.694)
  line L4354 (112.926, -109.958) -> (112.953, -110.011)
  line L4355 (113.277, -109.607) -> (112.926, -109.958)
  line L4356 (112.953, -110.011) -> (112.973, -110.134)
  line L4357 (112.749, -109.781) -> (113.277, -109.253)
  line L4358 (124.148, -106.554) -> (124.131, -106.58)
  line L4359 (115.577, -108.267) -> (115.577, -108.34)
  line L4360 (114.277, -108.267) -> (114.277, -108.417)
  line L4361 (119.075, -110.233) -> (119.018, -110.344)
  line L4362 (124.352, -105.251) -> (124.409, -105.363)
  line L4363 (123.287, -107.406) -> (123.257, -107.415)
  line L4364 (124.263, -105.81) -> (124.153, -105.866)
  line L4365 (119.094, -110.109) -> (119.075, -110.233)
  line L4366 (123.328, -107.391) -> (123.325, -107.395)
  line L4367 (113.277, -108.267) -> (114.277, -108.267)
  line L4368 (114.277, -109.217) -> (114.577, -109.217)
  line L4369 (115.718, -108.204) -> (115.721, -108.2)
  line L4370 (112.173, -110.134) -> (112.192, -110.011)
  line L4371 (115.729, -108.196) -> (115.759, -108.189)
  line L4372 (123.346, -107.378) -> (123.328, -107.391)
  line L4373 (118.818, -109.729) -> (118.929, -109.785)
  line L4374 (118.641, -109.717) -> (118.694, -109.709)
  line L4375 (114.577, -108.817) -> (114.277, -108.817)
  line L4376 (124.409, -105.61) -> (124.352, -105.721)
  line L4377 (124.15, -106.541) -> (124.15, -106.545)
  line L4378 (124.149, -106.548) -> (124.148, -106.554)
  line L4379 (124.263, -105.163) -> (124.352, -105.251)
  line L4380 (112.696, -109.754) -> (112.749, -109.781)
  line L4381 (115.976, -108.181) -> (115.998, -108.184)
  line L4382 (112.249, -110.37) -> (112.192, -110.258)
  line L4383 (112.192, -110.011) -> (112.249, -109.899)
  line L4384 (113.277, -109.253) -> (113.277, -108.267)
  line L4385 (115.759, -108.189) -> (115.788, -108.181)
  line L4386 (112.338, -110.458) -> (112.249, -110.37)
  line L4387 (115.788, -108.181) -> (115.976, -108.181)
  line L4388 (124.152, -105.106) -> (124.263, -105.163)
  line L4389 (114.577, -108.417) -> (114.577, -108.267)
  line L4390 (112.573, -109.734) -> (112.696, -109.754)
  line L4391 (112.249, -109.899) -> (112.338, -109.811)
  line L4392 (112.192, -110.258) -> (112.173, -110.134)
  line L4393 (114.277, -108.817) -> (114.277, -109.217)
  line L4394 (115.723, -108.2) -> (115.729, -108.196)
  line L4395 (114.277, -108.417) -> (114.577, -108.417)
  line L4396 (114.577, -108.267) -> (115.577, -108.267)
  line L4397 (115.7, -108.217) -> (115.718, -108.204)
  line L4398 (123.322, -107.396) -> (123.317, -107.399)
  line L4399 (114.577, -109.217) -> (114.577, -108.817)
  line L4400 (118.694, -109.709) -> (118.818, -109.729)
  line L4401 (119.428, -107.173) -> (119.458, -107.165)
  line L4402 (123.903, -106.467) -> (123.903, -105.866)
  line L4403 (124.153, -105.866) -> (124.153, -106.519)
  line L4404 (119.018, -109.874) -> (119.075, -109.985)
  line L4405 (118.929, -110.433) -> (118.818, -110.489)
  line L4406 (118.428, -108.142) -> (119.369, -107.201)
  line L4407 (118.314, -109.985) -> (118.371, -109.874)
  line L4408 (123.648, -105.61) -> (123.628, -105.486)
  line L4409 (124.153, -106.519) -> (124.15, -106.541)
  line L4410 (124.131, -106.58) -> (124.117, -106.607)
  line L4411 (118.294, -110.109) -> (118.314, -109.985)
  line L4412 (118.929, -109.785) -> (119.018, -109.874)
  line L4413 (118.395, -108.209) -> (118.394, -108.204)
  line L4414 (124.428, -105.486) -> (124.409, -105.61)
  line L4415 (124.409, -105.363) -> (124.428, -105.486)
  line L4416 (118.371, -109.874) -> (118.391, -109.853)
  line L4417 (119.398, -107.18) -> (119.428, -107.173)
  line L4418 (124.15, -106.545) -> (124.149, -106.548)
  line L4419 (119.39, -107.184) -> (119.393, -107.184)
  line L4420 (118.694, -110.509) -> (118.571, -110.489)
  line L4421 (119.509, -107.415) -> (118.641, -108.283)
  line L4422 (123.205, -107.165) -> (123.903, -106.467)
  line L4423 (123.903, -105.866) -> (123.793, -105.81)
  line L4424 (118.459, -110.433) -> (118.371, -110.344)
  line L4425 (123.325, -107.395) -> (123.322, -107.396)
  line L4426 (123.317, -107.399) -> (123.287, -107.406)
  line L4427 (119.018, -110.344) -> (118.929, -110.433)
  line L4428 (118.391, -109.853) -> (118.391, -108.231)
  line L4429 (119.393, -107.184) -> (119.398, -107.18)
  line L4430 (118.641, -108.283) -> (118.641, -109.717)
  line L4431 (118.396, -108.202) -> (118.397, -108.195)
  line L4432 (124.117, -106.607) -> (123.346, -107.378)
  line L4433 (123.793, -105.81) -> (123.705, -105.721)
  line L4434 (124.352, -105.721) -> (124.263, -105.81)
  line L4435 (123.257, -107.415) -> (119.509, -107.415)
  line L4436 (118.397, -108.195) -> (118.413, -108.169)
  line L4437 (118.818, -110.489) -> (118.694, -110.509)
  line L4438 (118.394, -108.204) -> (118.396, -108.202)
  line L4439 (123.705, -105.721) -> (123.648, -105.61)
  line L4440 (119.369, -107.201) -> (119.387, -107.188)
  line L4441 (119.387, -107.188) -> (119.39, -107.184)
  line L4442 (119.075, -109.985) -> (119.094, -110.109)
  line L4443 (118.314, -110.233) -> (118.294, -110.109)
  line L4444 (133.79, -109.553) -> (133.81, -109.593)
  line L4445 (133.429, -109.317) -> (133.553, -109.336)
  line L4446 (135.734, -108.095) -> (135.853, -108.172)
  line L4447 (133.306, -109.336) -> (133.429, -109.317)